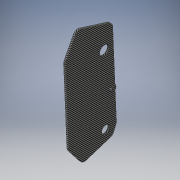
# Autodesk Inventor part: Module Plate 1
Saved by Autodesk Inventor 2019.4 (Build 234330000, 330)
## iProperties
Created: 2019-10-19
Part Number: Module Plate 1
Material: CFRP
Document SubType Name: Modeling
Designer: admin
Density: 1.43 g/cm^3
Appearance: Carbon Fiber
d27: 7.000 mm
Height: 80.000 mm
Author: admin
Autodesk Inventor part; units mm, degrees
ref_plane "YZ Plane" through (0, 0, 0) normal (1, 0, 0) x (0, 1, 0)
ref_plane "XZ Plane" through (0, 0, 0) normal (0, 1, 0) x (-1, 0, 0)
ref_plane "XY Plane" through (0, 0, 0) normal (0, 0, 1) x (1, 0, 0)
sketch "Sketch1" plane through (0, 0, 0) normal (1, 0, 0) x (0, 1, 0)
  circle A0 centre (0, 0) radius 62.5 construction
  circle A1 centre (-143.2302, -2.5) radius 50 construction
  line L0 (-143.2302, -2.5) -> (0, 0) construction
  line L1 (-172.7208, -52.5) -> (-113.4241, -52.5) construction
  line L2 (-16.0459, -62.5) -> (40.9165, -62.5) construction
  line L3 (-160.0196, -17.2687) -> (-141.4889, -24.7928)
  line L4 (-141.4889, -24.7928) -> (-81.8325, -22.1672)
  line L5 (41.9129, -16.7211) -> (64.9391, 56.3978)
  line L6 (64.9391, 56.3978) -> (17.8977, 80.8651)
  line L7 (17.8977, 80.8651) -> (-142.9104, 73.7878)
  line L8 (-142.9104, 73.7878) -> (-180.0842, 44.8475)
  line L9 (-180.0842, 44.8475) -> (-160.0196, -17.2687)
  circle A2 centre (0, 0) radius 9.8
  circle A3 centre (-143.2302, -2.5) radius 8.3
  line L10 (-150.7542, -21.0307) -> (-143.2302, -2.5) construction
  arc A4 (-81.8325, -22.1672) -> (-70.5297, -21.6698) centre (-76.4889, -14.9253) ccw
  arc A5 (-70.5297, -21.6698) -> (-81.8325, -22.1672) centre (-76.4889, -14.9253) ccw construction
  line L11 (-97.1128, -22.8397) -> (-96.4745, -22.8117) construction
  line L12 (-96.4745, -22.8117) -> (-70.5297, -21.6698) construction
  line L13 (-81.8325, -22.1672) -> (-97.1128, -22.8397) construction
  line L14 (-70.5297, -21.6698) -> (41.9129, -16.7211)
  circle A6 centre (-76.4889, -14.9253) radius 4
  line L15 (0, 0) -> (-212.6616, 0) construction
  dimension "d0" = 125
  dimension "d1" = 100
  dimension "d2" = 143.252
  dimension "d3" = 10
  dimension "d4" = 20
  dimension "d5" = 19.6
  dimension "d6" = 16.6
  dimension "d7" = 23.099
  dimension "d8" = 20
  dimension "d9" = 130
  dimension "d10" = 110
  dimension "d12" = 155.381
  dimension "d13" = 80
  dimension "d14" = 100
  dimension "d15" = 150
  dimension "Height" = 80
  dimension "d17" = 45
  dimension "d18" = 60
  dimension "d19" = 18
  dimension "d26" = 8
  dimension "d27" = 7
  dimension "d28" = 65
  constraints: 32 end point, 7 centre point, 5 parallel, 4 coincident, 4 point on circle, 3 horizontal, 2 point on line, 2 tangent, 1 midpoint, 1 perpendicular
  measures "d0" diameter of A0
  measures "d1" diameter of A1
  measures "d2" distance of L0.start L0.end
  measures "d3" distance between parallel lines of L2 L1
  measures "d4" distance from line of L0.start L3
  measures "d5" diameter of A2
  measures "d6" diameter of A3
  measures "d7" angle of L0 L3
  measures "d8" distance of L3.start L3.end
  measures "d9" angle of L3 L9
  measures "d10" angle of L9 L8
  measures "d12" angle of L4 L3
  measures "d13" distance from line of L15.start L7
  measures "d14" angle of L5 L6
  measures "d15" angle of L7 L6
  measures "Height" distance from line of point (0, 0) L6
  measures "d17" distance from line of L15.start L5
  measures "d18" distance from line of L10.end L8
  measures "d19" diameter of A4
  measures "d26" diameter of A6
  measures "d27" distance from line of L4 A6.centre
  measures "d28" horizontal distance of L3.end A6.centre
extrude "Extrusion1" add sketch "Sketch1" along normal blind 4
fillet "Fillet1" radius 2 2 edges at (2, -81.8325, -22.1672) (2, -70.5297, -21.6698)
fillet "Fillet2" radius 10 7 edges at (2, -180.0842, 44.8475) (2, -142.9104, 73.7878) (2, -160.0196, -17.2687) (2, 17.8977, 80.8651) (2, 64.9391, 56.3978) (2, 41.9129, -16.7211) (2, -141.4889, -24.7928)
body "Solid1"
